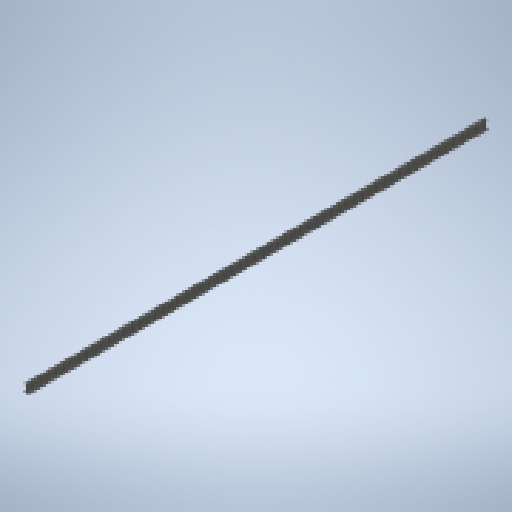
# Autodesk Inventor part: Long I-Beam
Saved by Autodesk Inventor 2025 (Build 290162000, 162)
## iProperties
Created: 2024-06-26
Part Number: Long I-Beam
Material: Steel ASTM A36
Document SubType Name: Modeling
Designer: track
Density: 7.85 g/cm^3
Appearance: Plate
Author: track
Autodesk Inventor part; units mm, degrees
ref_plane "YZ Plane" through (0, 0, 0) normal (1, 0, 0) x (0, 1, 0)
ref_plane "XZ Plane" through (0, 0, 0) normal (0, 1, 0) x (-1, 0, 0)
ref_plane "XY Plane" through (0, 0, 0) normal (0, 0, 1) x (1, 0, 0)
sketch "Sketch1" plane through (0, 0, 0) normal (0, 0, 1) x (1, 0, 0)
  line L0 (0, 0) -> (-50.8, -19.05)
  line L1 (76.2, -19.05) -> (25.4, 0)
  line L2 (25.4, 0) -> (25.4, 127)
  line L3 (25.4, 127) -> (50.8, 142.875)
  line L4 (-25.4, 142.875) -> (0, 127)
  line L5 (0, 127) -> (0, 0)
  line L6 (0, 0) -> (25.4, 0) construction
  line L7 (0, 127) -> (25.4, 127) construction
  line L8 (12.7, 0) -> (12.7, 127) construction
  line L9 (-50.8, -19.05) -> (-50.8, -25.4)
  line L10 (-50.8, -25.4) -> (76.2, -25.4)
  line L11 (76.2, -25.4) -> (76.2, -19.05)
  line L12 (50.8, 142.875) -> (50.8, 152.4)
  line L13 (50.8, 152.4) -> (-25.4, 152.4)
  line L14 (-25.4, 142.875) -> (50.8, 142.875) construction
  line L15 (-50.8, -19.05) -> (76.2, -19.05) construction
  line L16 (-25.4, 142.875) -> (-25.4, 152.4)
  line L17 (0, 0) -> (12.7, 0) construction
  line L18 (12.7, 0) -> (12.7, 152.4) construction
  line L19 (12.7, 152.4) -> (50.8, 152.4)
  dimension "d1" = 127
  dimension "d2" = 15.875
  dimension "d3" = 25.4
  dimension "d4" = 6.35
  dimension "d8" = 50.8
  dimension "d9" = 50.8
  dimension "d10" = 25.4
  dimension "d11" = 127
  dimension "d12" = 25.4
  dimension "d13" = 177.8
  dimension "d14" = 25.4
  dimension "d17" = 12.7
  constraints: 40 end point, 4 perpendicular, 4 vertical, 3 midpoint, 2 horizontal, 1 collinear, 1 parallel
  measures "d1" distance of L1.end L2.end
  measures "d2" vertical distance of L2.end L3.end
  measures "d3" horizontal distance of L2.end L3.end
  measures "d4" distance of L10.end L1.start
  measures "d8" horizontal distance of L1.start L1.end
  measures "d9" horizontal distance of L0.start L0.end
  measures "d10" distance from line of L10 L1.end
  measures "d11" distance of L9.end L10.end
  measures "d12" horizontal distance of L4.start L4.end
  measures "d13" distance between parallel lines of L13 L10
  measures "d14" distance from line of L2 L0.start
  measures "d17" distance from line of L0.start L8
extrude "Extrusion1" add sketch "Sketch1" against normal blind 10560.05
body "Solid1"
